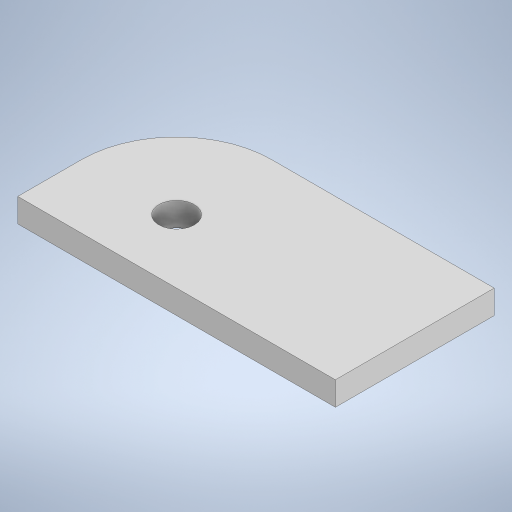
# Autodesk Inventor part: PovorotBlockOsnova
Saved by Autodesk Inventor 2024 (Build 280153000, 153)
## iProperties
Created: 2023-11-12
Part Number: PovorotBlockOsnova
Material: Generic
Document SubType Name: Modeling
Designer: KirikDK
Density: 1 g/cm^3
Appearance: Default
Author: KirikDK
Autodesk Inventor part; units mm, degrees
ref_plane "YZ Plane" through (0, 0, 0) normal (1, 0, 0) x (0, 1, 0)
ref_plane "XZ Plane" through (0, 0, 0) normal (0, 1, 0) x (-1, 0, 0)
ref_plane "XY Plane" through (0, 0, 0) normal (0, 0, 1) x (1, 0, 0)
sketch "Sketch1" plane through (0, 0, 0) normal (0, 1, 0) x (-1, 0, 0)
  line L0 (176.8421, 47.7193) -> (-23.1579, 47.7193)
  line L1 (-23.1579, 47.7193) -> (-23.1579, -52.2807)
  line L2 (-23.1579, -52.2807) -> (176.8421, -52.2807)
  line L3 (176.8421, -52.2807) -> (176.8421, 47.7193)
  point P0 (0, 0)
  dimension "d0" = 100
  dimension "d1" = 200
  constraints: 8 end point, 2 parallel, 1 horizontal, 1 perpendicular
  measures "d0" distance of L2.end L0.start
  measures "d1" distance of L0.start L0.end
extrude "Extrusion1" add sketch "Sketch1" along normal blind 15
fillet "Fillet2" radius 60 1 edges at (-176.8421, 7.5, -52.2807)
sketch "Sketch2" plane through (0, 15, 0) normal (0, 1, 0) x (1, 0, 0)
  arc A0 (-116.8421, 52.2807) -> (-176.8421, -7.7193) centre (-116.8421, -7.7193) ccw projected
  circle A1 centre (-116.8421, -7.7193) radius 11.1579
  point P0 (0, 0)
  constraints: 1 centre point, 1 coincident
extrude "Extrusion2" cut sketch "Sketch2" against normal blind 15
body "Solid1"
